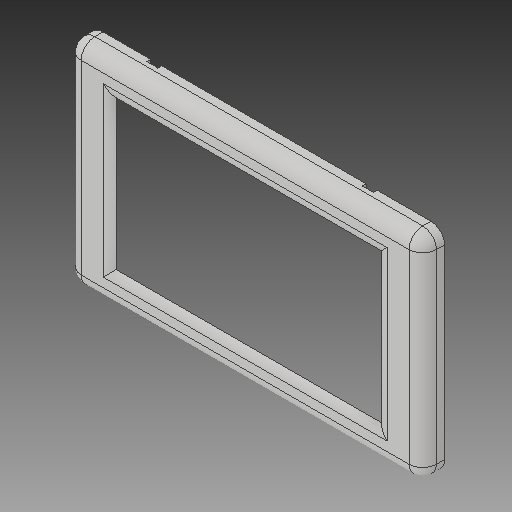
# Autodesk Inventor part: Better designed front piece
Saved by Autodesk Inventor 2018 (Build 220112000, 112)
## iProperties
Created: 2019-09-14
Part Number: Better designed front piece
Material: Generic
Document SubType Name: Modeling
Designer: Jacob
Density: 1 g/cm^3
Appearance: Default
Mass: 58.3028 g
Surface Area: 376.826 cm^2
Volume: 58.3028 cm^3
Author: Jacob
Autodesk Inventor part; units mm, degrees
ref_plane "YZ Plane" through (0, 0, 0) normal (1, 0, 0) x (0, 1, 0)
ref_plane "XZ Plane" through (0, 0, 0) normal (0, 1, 0) x (-1, 0, 0)
ref_plane "XY Plane" through (0, 0, 0) normal (0, 0, 1) x (1, 0, 0)
sketch "Sketch1" plane through (0, 0, 0) normal (0, 0, 1) x (1, 0, 0)
  line L0 (-97.5, 56) -> (97.5, 56)
  line L1 (97.5, 56) -> (97.5, -56)
  line L2 (97.5, -56) -> (-97.5, -56)
  line L3 (-97.5, -56) -> (-97.5, 56)
  line L4 (-97.5, 56) -> (97.5, -56) construction
  line L5 (97.5, 56) -> (-97.5, -56) construction
  point P0 (0, 0)
  dimension "d0" = 195
  dimension "d1" = 112
  constraints: 12 end point, 2 midpoint, 2 parallel, 1 horizontal, 1 perpendicular
  measures "d0" distance of L0.start L0.end
  measures "d1" distance of L0.end L1.end
extrude "Extrusion1" add sketch "Sketch1" against normal blind 9.9
shell "Shell1" thickness 6.35 outward yes removed faces 1 at (-32.5, 18.6667, -9.9)
fillet "Fillet1" radius 8 4 edges at (-103.85, 62.35, -1.775) (103.85, 62.35, -1.775) (103.85, -62.35, -1.775) (-103.85, -62.35, -1.775)
sketch "Sketch2" plane through (0, 0, 6.35) normal (0, 0, 1) x (1, 0, 0)
  line L0 (-77.5, 43.5) -> (77.5, 43.5)
  line L1 (77.5, 43.5) -> (77.5, -43.5)
  line L2 (77.5, -43.5) -> (-77.5, -43.5)
  line L3 (-77.5, -43.5) -> (-77.5, 43.5)
  line L4 (-77.5, 43.5) -> (77.5, -43.5) construction
  line L5 (77.5, 43.5) -> (-77.5, -43.5) construction
  point P0 (0, 0)
  dimension "d6" = 155
  dimension "d7" = 87
  constraints: 12 end point, 2 midpoint, 2 parallel, 1 horizontal, 1 perpendicular
  measures "d6" distance of L0.start L0.end
  measures "d7" distance of L0.end L1.end
extrude "Extrusion2" cut sketch "Sketch2" against normal blind 6.35
sketch "Sketch3" plane through (97.5, 56, 0) normal (0, 0, -1) x (-1, 0, 0)
  line L0 (195, 0) -> (0, 0) projected
  line L1 (0, -112) -> (195, -112)
  line L2 (195, -112) -> (195, 0)
  line L3 (195, 0) -> (0, 0)
  line L4 (0, 0) -> (0, -112)
  line L5 (0, -112) -> (195, 0) construction
  line L6 (195, -112) -> (0, 0) construction
  point P0 (97.5, -56)
  constraints: 12 end point, 2 midpoint, 2 parallel, 1 horizontal, 1 perpendicular
extrude "Extrusion3" cut sketch "Sketch3" against normal blind 3.175
sketch "Sketch4" plane through (0, 0, -9.9) normal (0, 0, -1) x (-1, 0, 0)
  line L0 (-97.5, -56) -> (-97.5, 56) projected
  line L1 (-97.5, 56) -> (-97.5, 62.178) construction
  arc A0 (-95.85, 62.35) -> (-103.85, 54.35) centre (-95.85, 54.35) ccw projected
  line L2 (-97.5, 56) -> (97.5, 56) projected
  line L3 (-97.5, 56) -> (-103.742, 56) construction
  line L4 (-97.5, 56) -> (-101.5069, 60.0069) construction
  circle A1 centre (-99.5034, 58.0034) radius 1
  line L5 (97.5, 56) -> (97.5, -56) projected
  line L6 (97.5, 56) -> (97.5, 62.178) construction
  line L7 (97.5, 56) -> (103.6959, 56) construction
  line L8 (97.5, 56) -> (101.5069, 60.0069) construction
  arc A2 (103.85, 54.35) -> (95.85, 62.35) centre (95.85, 54.35) ccw projected
  circle A3 centre (99.5034, 58.0034) radius 1
  line L9 (-97.5, -56) -> (-103.742, -56) construction
  line L10 (-97.5, -56) -> (-97.5, -62.1209) construction
  line L11 (-97.5, -56) -> (-101.5069, -60.0069) construction
  arc A4 (-103.85, -54.35) -> (-95.85, -62.35) centre (-95.85, -54.35) ccw projected
  circle A5 centre (-99.5034, -58.0034) radius 1
  line L12 (97.5, -56) -> (103.6959, -56) construction
  line L13 (97.5, -56) -> (97.5, -62.178) construction
  arc A6 (95.85, -62.35) -> (103.85, -54.35) centre (95.85, -54.35) ccw projected
  line L14 (97.5, -56) -> (101.5069, -60.0069) construction
  circle A7 centre (99.5034, -58.0034) radius 1
  line L15 (97.5, 0) -> (103.8479, 0) construction
  circle A8 centre (100.674, 0) radius 1
  line L16 (0, 56) -> (0, 62.8523) construction
  circle A9 centre (0, 59.4261) radius 1
  line L17 (97.5, -56) -> (-97.5, -56) projected
  line L18 (0, -56) -> (0, -62.8523) construction
  circle A10 centre (0, -59.4262) radius 1
  line L19 (-97.5, 0) -> (-103.85, 0) construction
  line L20 (-103.85, 54.35) -> (-103.85, -54.35) projected
  circle A11 centre (-100.675, 0) radius 1
  point P0 (0, 0)
  dimension "d22" = 2
  dimension "d23" = 2
  dimension "d24" = 2
  dimension "d25" = 2
  dimension "d26" = 2
  dimension "d27" = 2
  dimension "d28" = 2
  dimension "d29" = 2
  constraints: 32 end point, 13 midpoint, 8 centre point, 6 point on circle, 6 vertical, 5 horizontal
  measures "d22" diameter of A1
  measures "d23" diameter of A3
  measures "d24" diameter of A5
  measures "d25" diameter of A7
  measures "d26" diameter of A8
  measures "d27" diameter of A9
  measures "d28" diameter of A10
  measures "d29" diameter of A11
extrude "Extrusion4" [suppressed]
sketch "Sketch5" plane through (-97.5, -56, -9.9) normal (0, 1, 0) x (1, 0, 0)
  line L0 (0, -13.075) -> (195, -13.075) projected
  line L1 (0, 0) -> (0, -13.075) projected
  line L2 (195, -13.075) -> (0, -13.075)
  line L3 (0, -13.075) -> (0, -4.575)
  line L4 (0, -4.575) -> (195, -4.575) construction
  line L5 (195, -4.575) -> (195, -13.075)
  line L6 (163, -4.575) -> (163, -13.075) construction
  line L7 (35, -13.075) -> (35, -4.575) construction
  line L8 (0, 0) -> (195, 0) projected
  line L9 (163, -4.575) -> (163, 0)
  line L10 (35, -4.575) -> (35, 0) construction
  line L11 (159.9458, -4.575) -> (166.0458, -4.575)
  line L12 (166.0458, -4.575) -> (166.0458, -3.325)
  line L13 (166.0458, -3.325) -> (159.9458, -3.325)
  line L14 (159.9458, -3.325) -> (159.9458, -4.575)
  line L15 (38.05, -4.575) -> (31.95, -4.575)
  line L16 (31.95, -4.575) -> (31.95, -3.325)
  line L17 (31.95, -3.325) -> (38.05, -3.325)
  line L18 (38.05, -3.325) -> (38.05, -4.575)
  line L19 (38.05, -4.575) -> (31.95, -3.325) construction
  line L20 (31.95, -4.575) -> (38.05, -3.325) construction
  point P0 (97.5, -9.9)
  point P1 (163, -2.2875)
  point P2 (35, -3.95)
  dimension "d32" = 8.5
  dimension "d33" = 32
  dimension "d34" = 35
  dimension "d35" = 1.25
  dimension "d36" = 6.1
  dimension "d37" = 0
  dimension "d38" = 1.25
  dimension "d39" = 6.1
  dimension "d40" = 0
  constraints: 36 end point, 8 point on line, 6 parallel, 6 perpendicular, 3 horizontal, 3 midpoint, 1 vertical
  measures "d32" distance between parallel lines of L4 L0
  measures "d33" distance between parallel lines of L6 L5
  measures "d34" distance between parallel lines of L7 L3
  measures "d35" distance of L11.end L12.end
  measures "d36" distance of L12.end L13.end
  measures "d37" distance between parallel lines of L4 L11
  measures "d38" distance of L15.end L16.end
  measures "d39" distance of L16.end L17.end
  measures "d40" distance between parallel lines of L4 L15
extrude "Extrusion5" [suppressed]
sketch "Sketch6" plane through (0, 0, -9.9) normal (0, 0, -1) x (-1, 0, 0)
  line L0 (-130.7593, 67.2756) -> (130.7593, 67.2756)
  line L1 (130.7593, 67.2756) -> (130.7593, -67.2756)
  line L2 (130.7593, -67.2756) -> (-130.7593, -67.2756)
  line L3 (-130.7593, -67.2756) -> (-130.7593, 67.2756)
  line L4 (-130.7593, 67.2756) -> (130.7593, -67.2756) construction
  line L5 (130.7593, 67.2756) -> (-130.7593, -67.2756) construction
  point P0 (0, 0)
  constraints: 12 end point, 2 midpoint, 2 parallel, 1 horizontal, 1 perpendicular
extrude "Extrusion6" cut sketch "Sketch6" against normal blind 2.4638
sketch "Sketch7" plane through (0, 0, -7.4362) normal (0, 0, -1) x (-1, 0, 0)
  line L0 (95.85, -62.35) -> (-95.85, -62.35) projected
  line L1 (-61.25, -62.35) -> (-61.25, 62.35) construction
  line L2 (-95.85, 62.35) -> (95.85, 62.35) projected
  line L3 (-97.5, 56) -> (-97.5, -56) projected
  line L4 (64.75, -62.35) -> (64.75, 62.35) construction
  line L5 (97.5, -56) -> (97.5, 56) projected
  line L6 (-64.5, -62.35) -> (-58, -62.35)
  line L7 (-58, -62.35) -> (-58, 62.35)
  line L8 (-58, 62.35) -> (-64.5, 62.35)
  line L9 (-64.5, 62.35) -> (-64.5, -62.35)
  line L10 (-64.5, -62.35) -> (-58, 62.35) construction
  line L11 (-58, -62.35) -> (-64.5, 62.35) construction
  line L12 (61.5, -62.35) -> (68, -62.35)
  line L13 (68, -62.35) -> (68, 62.35)
  line L14 (68, 62.35) -> (61.5, 62.35)
  line L15 (61.5, 62.35) -> (61.5, -62.35)
  line L16 (61.5, -62.35) -> (68, 62.35) construction
  line L17 (68, -62.35) -> (61.5, 62.35) construction
  point P0 (0, 0)
  point P1 (-61.25, 0)
  point P2 (64.75, 0)
  dimension "d47" = 6.5
  dimension "d48" = 6.5
  dimension "d57" = 126
  dimension "d58" = 32.75
  constraints: 28 end point, 6 midpoint, 6 point on line, 4 parallel, 3 perpendicular, 2 horizontal, 1 vertical
  measures "d47" distance between parallel lines of L7 L9
  measures "d48" distance between parallel lines of L13 L15
  measures "d57" distance between parallel lines of L4 L1
  measures "d58" distance between parallel lines of L5 L4
extrude "Extrusion7" cut sketch "Sketch7" against normal blind 2.2 contours L0 L15 L2 L13 | L0 L9 L2 L7
sketch "Sketch9" plane through (0, 0, -5.2362) normal (0, 0, -1) x (-1, 0, 0)
  line L0 (-64.5, 56) -> (-64.5, 62.35) projected
  line L1 (-64.5, 59.175) -> (-58, 59.175) construction
  line L2 (-58, 62.35) -> (-58, 56) projected
  line L3 (-95.85, 62.35) -> (95.85, 62.35) projected
  line L4 (68, 62.35) -> (68, 56) projected
  line L5 (68, 59.175) -> (61.5, 59.175) construction
  line L6 (61.5, 56) -> (61.5, 62.35) projected
  line L7 (-64.5, -62.35) -> (-64.5, -56) projected
  line L8 (-64.5, -59.175) -> (-58, -59.175) construction
  line L9 (61.5, -62.35) -> (61.5, -56) projected
  line L10 (61.5, -59.175) -> (68, -59.175) construction
  line L11 (97.5, -56) -> (-97.5, -56) projected
  line L12 (68, -56) -> (68, -62.35) projected
  line L13 (-58, -56) -> (-58, -62.35) projected
  line L14 (-61.25, 59.175) -> (-61.25, 56) construction
  line L15 (-61.25, 59.175) -> (-61.25, 62.35) construction
  line L16 (-64.5, 62.35) -> (-58, 62.35) projected
  circle A0 centre (-61.25, 59.175) radius 1.5
  line L17 (64.75, 59.175) -> (64.75, 62.35) construction
  line L18 (64.75, 59.175) -> (64.75, 56) construction
  circle A1 centre (64.75, 59.175) radius 1.5
  line L19 (-61.25, -59.175) -> (-61.25, -56) construction
  line L20 (-61.25, -59.175) -> (-61.25, -62.35) construction
  line L21 (-58, -62.35) -> (-64.5, -62.35) projected
  circle A2 centre (-61.25, -59.175) radius 1.5
  line L22 (64.75, -59.175) -> (64.75, -56) construction
  line L23 (64.75, -59.175) -> (64.75, -62.35) construction
  circle A3 centre (64.75, -59.175) radius 1.5
  point P0 (0, 0)
  dimension "d69" = 3
  dimension "d70" = 3
  dimension "d71" = 3
  dimension "d72" = 3
  constraints: 24 end point, 12 midpoint, 4 centre point, 4 coincident, 4 point on line, 4 vertical, 2 horizontal, 1 perpendicular
  measures "d69" diameter of A0
  measures "d70" diameter of A1
  measures "d71" diameter of A2
  measures "d72" diameter of A3
extrude "Extrusion10" cut sketch "Sketch9" against normal blind 3 contours A0 | A1 | A2 | A3
sketch "Sketch10" plane through (0, 0, 6.35) normal (0, 0, 1) x (1, 0, 0)
  line L0 (-169.0773, 99.7434) -> (160.0413, 99.7434)
  line L1 (160.0413, 99.7434) -> (160.0413, -85.1468)
  line L2 (160.0413, -85.1468) -> (-169.0773, -85.1468)
  line L3 (-169.0773, -85.1468) -> (-169.0773, 99.7434)
  point P0 (0, 0)
  constraints: 8 end point, 2 parallel, 1 horizontal, 1 perpendicular
extrude "Extrusion11" cut sketch "Sketch10" against normal blind 1
fillet "Fillet6" radius 8 8 edges at (101.5069, -60.0069, 5.35) (0, -62.35, 5.35) (-101.5069, -60.0069, 5.35) (-103.85, 0, 5.35) (-101.5069, 60.0069, 5.35) (0, 62.35, 5.35) (101.5069, 60.0069, 5.35) (103.85, 0, 5.35)
fillet "Fillet7" radius 8 4 edges at (-77.5, 0, 5.35) (0, 43.5, 5.35) (0, -43.5, 5.35) (77.5, 0, 5.35)
body "Solid1"
